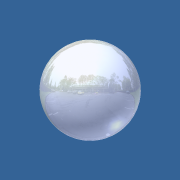
# Autodesk Inventor part: 2009_CTS_Light
Saved by Autodesk Inventor 2012 (Build 160160000, 160)
## iProperties
Company: Team 801
Created: 2009-01-31
Part Number: 2009_CTS_Light
Document SubType Name: Modeling
Designer: Jeffrey M
Density: 1 g/cm^3
Description: Reciever Light
Material: Default
Title: 2009_CTS_Light
Author: Jeffrey M
Autodesk Inventor part; units mm, degrees
ref_plane "YZ Plane" through (0, 0, 0) normal (1, 0, 0) x (0, 1, 0)
ref_plane "XZ Plane" through (0, 0, 0) normal (0, 1, 0) x (-1, 0, 0)
ref_plane "XY Plane" through (0, 0, 0) normal (0, 0, 1) x (1, 0, 0)
sketch "Sketch1" plane through (0, 0, 0) normal (0, 0, 1) x (1, 0, 0)
  arc A0 (0, -2.413) -> (0, 2.7686) centre (0, 0.1778) ccw
  line L0 (0, 2.7686) -> (0, -2.413)
  dimension "d0" = 5.1816
  dimension "d0" = 5.1816
  constraints: 2 end point, 2 point on circle, 1 centre point, 1 vertical
  measures "d0" diameter of A0
revolve "Revolution1" add sketch "Sketch1" angle 360 about axis through (0, 2.7686, 0) along (0, -1, 0)
body "Solid1"
